Autodesk Inventor part; units mm, degrees
(part 2 of 2)
  arc A28 (126.7323, -21.9876) -> (127.2532, -22.5367) centre (141.5, -8.5) ccw projected
  spline S25 degree 3 poles (129.1537, -24.2343) (129.1768, -24.1247) (129.2231, -23.9054) (129.3093, -23.5804) (129.3922, -23.3127) (129.4667, -23.1013) (129.5266, -22.9443) (129.5917, -22.7893) (129.6822, -22.5842) (129.7847, -22.4159) (129.8454, -22.2589) (129.8618, -22.1906) (129.8689, -22.135) (129.8697, -22.0929) (129.8675, -22.0509) (129.8611, -22.0093) (129.8504, -21.9686) (129.8355, -21.9293) (129.8175, -21.8911) (129.7936, -21.8565) (129.7686, -21.8226) (129.728, -21.7839) (129.675, -21.7381) (129.6236, -21.6906) (129.5805, -21.6546) (129.544, -21.6335) (129.5069, -21.6137) (129.467, -21.6001) (129.4263, -21.5897) (129.3846, -21.5837) (129.3426, -21.5819) (129.3006, -21.5846) (129.2589, -21.5901) (129.2044, -21.6033) (129.1384, -21.6273) (128.9892, -21.7053) (128.8335, -21.826) (128.6398, -21.9391) (128.4932, -22.0211) (128.3438, -22.0983) (128.1422, -22.1961) (127.8855, -22.3086) (127.5723, -22.4308) (127.3595, -22.5014) (127.2532, -22.5367) knots 0 0 0 0 0.033613 0.067227 0.100839 0.117647 0.134454 0.151261 0.168068 0.201677 0.210077 0.218473 0.222676 0.226878 0.231076 0.235279 0.239479 0.24368 0.247882 0.252083 0.256283 0.260485 0.268889 0.277292 0.281494 0.285694 0.289895 0.294097 0.298298 0.302498 0.306701 0.310899 0.315101 0.319304 0.3277 0.3361 0.369709 0.386516 0.403323 0.420131 0.436938 0.470551 0.504164 0.537777 0.537777 0.537777 0.537777 projected
  arc A29 (129.1537, -24.2343) -> (129.7579, -24.6902) centre (141.5, -8.5) ccw projected
  spline S26 degree 3 poles (131.9119, -26.0519) (131.9167, -25.9399) (131.9262, -25.716) (131.9577, -25.3812) (131.9954, -25.1035) (132.0341, -24.8828) (132.0674, -24.718) (132.106, -24.5544) (132.1616, -24.3372) (132.235, -24.1544) (132.269, -23.9895) (132.274, -23.9194) (132.2718, -23.8634) (132.2656, -23.8218) (132.2566, -23.7807) (132.2434, -23.7408) (132.2262, -23.7023) (132.205, -23.666) (132.181, -23.6314) (132.1517, -23.6012) (132.1215, -23.5719) (132.075, -23.5403) (132.0152, -23.5039) (131.9567, -23.4655) (131.9082, -23.4371) (131.8688, -23.4223) (131.8289, -23.4088) (131.7873, -23.402) (131.7454, -23.3984) (131.7033, -23.3994) (131.6616, -23.4046) (131.6206, -23.4141) (131.5804, -23.4263) (131.5288, -23.4484) (131.4676, -23.4829) (131.3333, -23.5844) (131.1996, -23.7291) (131.0272, -23.8725) (130.8961, -23.9776) (130.7615, -24.0783) (130.5787, -24.2079) (130.344, -24.3611) (130.0551, -24.5332) (129.857, -24.6379) (129.7579, -24.6902) knots 0 0 0 0 0.033613 0.067227 0.100839 0.117647 0.134454 0.151261 0.168068 0.201677 0.210077 0.218473 0.222676 0.226878 0.231076 0.235279 0.239479 0.24368 0.247882 0.252083 0.256283 0.260485 0.268889 0.277292 0.281494 0.285694 0.289895 0.294097 0.298298 0.302498 0.306701 0.310899 0.315101 0.319304 0.3277 0.3361 0.369709 0.386516 0.403323 0.420131 0.436938 0.470551 0.504164 0.537777 0.537777 0.537777 0.537777 projected
  arc A30 (131.9119, -26.0519) -> (132.5828, -26.4021) centre (141.5, -8.5) ccw projected
  spline S27 degree 3 poles (134.9316, -27.3906) (134.9179, -27.2794) (134.8904, -27.057) (134.8664, -26.7216) (134.8579, -26.4415) (134.8597, -26.2174) (134.8654, -26.0494) (134.8766, -25.8817) (134.8957, -25.6583) (134.9379, -25.4659) (134.9444, -25.2976) (134.9378, -25.2277) (134.9264, -25.1728) (134.9134, -25.1328) (134.8978, -25.0937) (134.8782, -25.0565) (134.8549, -25.0214) (134.828, -24.9891) (134.7986, -24.9589) (134.7648, -24.9339) (134.7301, -24.91) (134.6791, -24.8865) (134.6141, -24.8604) (134.5501, -24.8322) (134.4976, -24.8121) (134.4563, -24.804) (134.4147, -24.7973) (134.3726, -24.7974) (134.3307, -24.8008) (134.2893, -24.8086) (134.249, -24.8206) (134.2101, -24.8368) (134.1725, -24.8555) (134.1252, -24.8857) (134.0706, -24.9298) (133.9548, -25.0521) (133.8467, -25.2168) (133.7003, -25.3866) (133.5882, -25.5118) (133.472, -25.6333) (133.3131, -25.7913) (133.1068, -25.981) (132.8502, -26.1983) (132.672, -26.3341) (132.5828, -26.4021) knots 0 0 0 0 0.033613 0.067227 0.100839 0.117647 0.134454 0.151261 0.168068 0.201677 0.210077 0.218473 0.222676 0.226878 0.231076 0.235279 0.239479 0.24368 0.247882 0.252083 0.256283 0.260485 0.268889 0.277292 0.281494 0.285694 0.289895 0.294097 0.298298 0.302498 0.306701 0.310899 0.315101 0.319304 0.3277 0.3361 0.369709 0.386516 0.403323 0.420131 0.436938 0.470551 0.504164 0.537777 0.537777 0.537777 0.537777 projected
  arc A31 (134.9316, -27.3906) -> (135.651, -27.6256) centre (141.5, -8.5) ccw projected
  spline S28 degree 3 poles (138.1305, -28.2141) (138.0986, -28.1067) (138.0349, -27.8918) (137.956, -27.5649) (137.9016, -27.29) (137.8665, -27.0687) (137.8445, -26.902) (137.8279, -26.7348) (137.8099, -26.5113) (137.8199, -26.3145) (137.7986, -26.1475) (137.7806, -26.0797) (137.7603, -26.0274) (137.7409, -25.99) (137.7191, -25.9541) (137.6936, -25.9206) (137.6648, -25.8898) (137.633, -25.8623) (137.5991, -25.8374) (137.5616, -25.8183) (137.5234, -25.8004) (137.4692, -25.7857) (137.4009, -25.7707) (137.333, -25.7534) (137.278, -25.7422) (137.2359, -25.741) (137.1938, -25.7412) (137.1523, -25.7482) (137.1115, -25.7585) (137.072, -25.773) (137.0342, -25.7915) (136.9985, -25.8138) (136.9644, -25.8385) (136.9228, -25.8761) (136.8762, -25.9286) (136.7821, -26.0682) (136.7026, -26.2485) (136.5861, -26.4401) (136.4962, -26.582) (136.4016, -26.721) (136.2708, -26.903) (136.0986, -27.1241) (135.8812, -27.3806) (135.7278, -27.544) (135.651, -27.6256) knots 0 0 0 0 0.033613 0.067227 0.100839 0.117647 0.134454 0.151261 0.168068 0.201677 0.210077 0.218473 0.222676 0.226878 0.231076 0.235279 0.239479 0.24368 0.247882 0.252083 0.256283 0.260485 0.268889 0.277292 0.281494 0.285694 0.289895 0.294097 0.298298 0.302498 0.306701 0.310899 0.315101 0.319304 0.3277 0.3361 0.369709 0.386516 0.403323 0.420131 0.436938 0.470551 0.504164 0.537777 0.537777 0.537777 0.537777 projected
  arc A32 (138.1305, -28.2141) -> (138.8788, -28.3275) centre (141.5, -8.5) ccw projected
  spline S29 degree 3 poles (141.4213, -28.4998) (141.3722, -28.3991) (141.274, -28.1976) (141.1424, -27.8882) (141.0434, -27.6261) (140.9724, -27.4135) (140.9232, -27.2527) (140.8793, -27.0905) (140.8248, -26.873) (140.8023, -26.6773) (140.7538, -26.5161) (140.7248, -26.4521) (140.6962, -26.4039) (140.6709, -26.3702) (140.6435, -26.3384) (140.6129, -26.3095) (140.5794, -26.2839) (140.5435, -26.262) (140.5059, -26.243) (140.4658, -26.2304) (140.4252, -26.219) (140.3693, -26.2134) (140.2994, -26.2098) (140.2297, -26.2039) (140.1735, -26.2019) (140.1318, -26.2077) (140.0904, -26.2148) (140.0505, -26.2286) (140.012, -26.2455) (139.9754, -26.2663) (139.9412, -26.2907) (139.9097, -26.3186) (139.8801, -26.3485) (139.8453, -26.3925) (139.8079, -26.452) (139.7381, -26.6052) (139.6893, -26.7961) (139.606, -27.0042) (139.5406, -27.159) (139.4702, -27.3117) (139.3711, -27.5127) (139.2377, -27.7591) (139.0655, -28.0479) (138.941, -28.2343) (138.8788, -28.3275) knots 0 0 0 0 0.033613 0.067227 0.100839 0.117647 0.134454 0.151261 0.168068 0.201677 0.210077 0.218473 0.222676 0.226878 0.231076 0.235279 0.239479 0.24368 0.247882 0.252083 0.256283 0.260485 0.268889 0.277292 0.281494 0.285694 0.289895 0.294097 0.298298 0.302498 0.306701 0.310899 0.315101 0.319304 0.3277 0.3361 0.369709 0.386516 0.403323 0.420131 0.436938 0.470551 0.504164 0.537777 0.537777 0.537777 0.537777 projected
  arc A33 (141.4213, -28.4998) -> (142.178, -28.4885) centre (141.5, -8.5) ccw projected
  spline S30 degree 3 poles (144.7142, -28.24) (144.6492, -28.1488) (144.5192, -27.9662) (144.3384, -27.6826) (144.1977, -27.4404) (144.0926, -27.2424) (144.0177, -27.0919) (143.9477, -26.9391) (143.8581, -26.7336) (143.8037, -26.5442) (143.7293, -26.3932) (143.6902, -26.3348) (143.654, -26.292) (143.6236, -26.2629) (143.5913, -26.236) (143.5563, -26.2126) (143.5191, -26.1929) (143.4801, -26.1772) (143.4399, -26.1646) (143.3982, -26.1588) (143.3563, -26.1542) (143.3003, -26.1579) (143.2307, -26.1659) (143.161, -26.1715) (143.1053, -26.1788) (143.0651, -26.1914) (143.0254, -26.2052) (142.9883, -26.2254) (142.9531, -26.2483) (142.9204, -26.2749) (142.8907, -26.3047) (142.8642, -26.3373) (142.84, -26.3717) (142.8128, -26.4208) (142.7858, -26.4856) (142.7421, -26.6482) (142.7255, -26.8446) (142.6775, -27.0636) (142.6385, -27.227) (142.5942, -27.3892) (142.5296, -27.6038) (142.4385, -27.8688) (142.3162, -28.182) (142.2241, -28.3863) (142.178, -28.4885) knots 0 0 0 0 0.033613 0.067227 0.100839 0.117647 0.134454 0.151261 0.168068 0.201677 0.210077 0.218473 0.222676 0.226878 0.231076 0.235279 0.239479 0.24368 0.247882 0.252083 0.256283 0.260485 0.268889 0.277292 0.281494 0.285694 0.289895 0.294097 0.298298 0.302498 0.306701 0.310899 0.315101 0.319304 0.3277 0.3361 0.369709 0.386516 0.403323 0.420131 0.436938 0.470551 0.504164 0.537777 0.537777 0.537777 0.537777 projected
  arc A34 (144.7142, -28.24) -> (145.4588, -28.1043) centre (141.5, -8.5) ccw projected
  spline S31 degree 3 poles (147.9195, -27.4418) (147.8403, -27.3624) (147.6821, -27.2038) (147.4571, -26.9538) (147.2784, -26.738) (147.1421, -26.56) (147.0434, -26.424) (146.9493, -26.2847) (146.8271, -26.0968) (146.7423, -25.9189) (146.644, -25.7822) (146.5958, -25.7311) (146.5531, -25.6948) (146.5183, -25.6711) (146.482, -25.6499) (146.4437, -25.6326) (146.4037, -25.6192) (146.3627, -25.6102) (146.3209, -25.6044) (146.2788, -25.6055) (146.2368, -25.6079) (146.1821, -25.6207) (146.1148, -25.6401) (146.047, -25.6571) (145.9932, -25.6735) (145.9557, -25.6925) (145.9187, -25.7127) (145.8855, -25.7387) (145.8546, -25.7671) (145.8267, -25.7987) (145.8023, -25.8329) (145.7815, -25.8695) (145.7633, -25.9074) (145.7446, -25.9603) (145.7286, -26.0287) (145.7123, -26.1963) (145.7282, -26.3927) (145.7169, -26.6166) (145.7054, -26.7842) (145.6883, -26.9515) (145.6599, -27.1738) (145.6137, -27.4501) (145.5446, -27.7792) (145.4874, -27.9959) (145.4588, -28.1043) knots 0 0 0 0 0.033613 0.067227 0.100839 0.117647 0.134454 0.151261 0.168068 0.201677 0.210077 0.218473 0.222676 0.226878 0.231076 0.235279 0.239479 0.24368 0.247882 0.252083 0.256283 0.260485 0.268889 0.277292 0.281494 0.285694 0.289895 0.294097 0.298298 0.302498 0.306701 0.310899 0.315101 0.319304 0.3277 0.3361 0.369709 0.386516 0.403323 0.420131 0.436938 0.470551 0.504164 0.537777 0.537777 0.537777 0.537777 projected
  arc A35 (147.9195, -27.4418) -> (148.6315, -27.1853) centre (141.5, -8.5) ccw projected
  spline S32 degree 3 poles (150.9496, -26.1268) (150.8585, -26.0616) (150.6763, -25.9311) (150.4132, -25.7216) (150.2014, -25.5382) (150.0378, -25.3851) (149.918, -25.2671) (149.8022, -25.1453) (149.6508, -24.98) (149.5378, -24.8185) (149.4184, -24.6998) (149.3625, -24.6574) (149.3144, -24.6286) (149.2761, -24.611) (149.2368, -24.596) (149.1962, -24.5852) (149.1546, -24.5786) (149.1126, -24.5765) (149.0705, -24.5776) (149.0291, -24.5856) (148.9881, -24.5949) (148.9362, -24.6166) (148.8731, -24.6467) (148.8089, -24.6747) (148.7586, -24.6997) (148.7247, -24.7247) (148.6916, -24.7506) (148.6631, -24.7817) (148.6372, -24.8149) (148.615, -24.8506) (148.5965, -24.8884) (148.5821, -24.9279) (148.5703, -24.9683) (148.5606, -25.0235) (148.556, -25.0936) (148.5675, -25.2616) (148.6155, -25.4527) (148.6413, -25.6754) (148.6575, -25.8427) (148.6682, -26.0104) (148.6768, -26.2344) (148.6767, -26.5146) (148.6627, -26.8506) (148.6419, -27.0737) (148.6315, -27.1853) knots 0 0 0 0 0.033613 0.067227 0.100839 0.117647 0.134454 0.151261 0.168068 0.201677 0.210077 0.218473 0.222676 0.226878 0.231076 0.235279 0.239479 0.24368 0.247882 0.252083 0.256283 0.260485 0.268889 0.277292 0.281494 0.285694 0.289895 0.294097 0.298298 0.302498 0.306701 0.310899 0.315101 0.319304 0.3277 0.3361 0.369709 0.386516 0.403323 0.420131 0.436938 0.470551 0.504164 0.537777 0.537777 0.537777 0.537777 projected
  arc A36 (150.9496, -26.1268) -> (151.6098, -25.7567) centre (141.5, -8.5) ccw projected
  spline S33 degree 3 poles (153.722, -24.331) (153.6214, -24.2817) (153.4202, -24.183) (153.1263, -24.0197) (152.8871, -23.8736) (152.7005, -23.7495) (152.563, -23.6528) (152.4287, -23.5517) (152.2521, -23.4136) (152.1141, -23.273) (151.9768, -23.1755) (151.9147, -23.1429) (151.8625, -23.1224) (151.8219, -23.1113) (151.7806, -23.103) (151.7387, -23.0991) (151.6966, -23.0994) (151.6549, -23.1042) (151.6135, -23.1123) (151.5741, -23.127) (151.5351, -23.1429) (151.4875, -23.1728) (151.4302, -23.2129) (151.3715, -23.2511) (151.326, -23.284) (151.2966, -23.3142) (151.2683, -23.3453) (151.2453, -23.3807) (151.2252, -23.4176) (151.2092, -23.4565) (151.1972, -23.4969) (151.1894, -23.5382) (151.1845, -23.58) (151.184, -23.636) (151.191, -23.7059) (151.23, -23.8697) (151.3088, -24.0503) (151.3709, -24.2657) (151.4144, -24.4281) (151.4526, -24.5918) (151.4979, -24.8113) (151.5439, -25.0877) (151.5854, -25.4214) (151.6017, -25.6449) (151.6098, -25.7567) knots 0 0 0 0 0.033613 0.067227 0.100839 0.117647 0.134454 0.151261 0.168068 0.201677 0.210077 0.218473 0.222676 0.226878 0.231076 0.235279 0.239479 0.24368 0.247882 0.252083 0.256283 0.260485 0.268889 0.277292 0.281494 0.285694 0.289895 0.294097 0.298298 0.302498 0.306701 0.310899 0.315101 0.319304 0.3277 0.3361 0.369709 0.386516 0.403323 0.420131 0.436938 0.470551 0.504164 0.537777 0.537777 0.537777 0.537777 projected
  arc A37 (153.722, -24.331) -> (154.3123, -23.8573) centre (141.5, -8.5) ccw projected
  spline S34 degree 3 poles (156.161, -22.1034) (156.0537, -22.0713) (155.839, -22.0071) (155.5221, -21.8944) (155.2622, -21.7897) (155.0578, -21.698) (154.9062, -21.6253) (154.7571, -21.5476) (154.5602, -21.4405) (154.4009, -21.3245) (154.2495, -21.251) (154.1828, -21.229) (154.1279, -21.2173) (154.086, -21.2131) (154.044, -21.2117) (154.002, -21.2147) (153.9606, -21.222) (153.9201, -21.2336) (153.8807, -21.2484) (153.8442, -21.2694) (153.8084, -21.2915) (153.7664, -21.3288) (153.7164, -21.3778) (153.6648, -21.4251) (153.6254, -21.4651) (153.6014, -21.4997) (153.5785, -21.535) (153.5617, -21.5737) (153.548, -21.6134) (153.5385, -21.6545) (153.5333, -21.6962) (153.5325, -21.7383) (153.5345, -21.7803) (153.5432, -21.8357) (153.5616, -21.9035) (153.6271, -22.0586) (153.7345, -22.2237) (153.8312, -22.426) (153.9008, -22.579) (153.9655, -22.7342) (154.0462, -22.9432) (154.1371, -23.2083) (154.233, -23.5306) (154.2858, -23.7484) (154.3123, -23.8573) knots 0 0 0 0 0.033613 0.067227 0.100839 0.117647 0.134454 0.151261 0.168068 0.201677 0.210077 0.218473 0.222676 0.226878 0.231076 0.235279 0.239479 0.24368 0.247882 0.252083 0.256283 0.260485 0.268889 0.277292 0.281494 0.285694 0.289895 0.294097 0.298298 0.302498 0.306701 0.310899 0.315101 0.319304 0.3277 0.3361 0.369709 0.386516 0.403323 0.420131 0.436938 0.470551 0.504164 0.537777 0.537777 0.537777 0.537777 projected
  arc A38 (156.161, -22.1034) -> (156.6652, -21.539) centre (141.5, -8.5) ccw projected
  spline S35 degree 3 poles (158.2001, -19.5048) (158.089, -19.4908) (157.8666, -19.4628) (157.5355, -19.4037) (157.262, -19.3432) (157.0452, -19.2864) (156.8837, -19.2397) (156.7239, -19.1876) (156.512, -19.1143) (156.3358, -19.0261) (156.1743, -18.9786) (156.1049, -18.9678) (156.0489, -18.9654) (156.0069, -18.9681) (155.9652, -18.9737) (155.9243, -18.9836) (155.8846, -18.9976) (155.8466, -19.0156) (155.8101, -19.0367) (155.7776, -19.0634) (155.7459, -19.0911) (155.7106, -19.1349) (155.6694, -19.1914) (155.6263, -19.2466) (155.594, -19.2925) (155.576, -19.3306) (155.5593, -19.3692) (155.549, -19.4101) (155.542, -19.4516) (155.5395, -19.4936) (155.5412, -19.5356) (155.5473, -19.5772) (155.5562, -19.6183) (155.5739, -19.6716) (155.6033, -19.7354) (155.6933, -19.8776) (155.8265, -20.0228) (155.9551, -20.2064) (156.049, -20.3458) (156.1383, -20.4883) (156.2524, -20.6812) (156.3857, -20.9277) (156.5333, -21.2298) (156.6213, -21.4359) (156.6652, -21.539) knots 0 0 0 0 0.033613 0.067227 0.100839 0.117647 0.134454 0.151261 0.168068 0.201677 0.210077 0.218473 0.222676 0.226878 0.231076 0.235279 0.239479 0.24368 0.247882 0.252083 0.256283 0.260485 0.268889 0.277292 0.281494 0.285694 0.289895 0.294097 0.298298 0.302498 0.306701 0.310899 0.315101 0.319304 0.3277 0.3361 0.369709 0.386516 0.403323 0.420131 0.436938 0.470551 0.504164 0.537777 0.537777 0.537777 0.537777 projected
  arc A39 (158.2001, -19.5048) -> (158.6046, -18.8651) centre (141.5, -8.5) ccw projected
  spline S36 degree 3 poles (159.7837, -16.6059) (159.6717, -16.6104) (159.4478, -16.6194) (159.1115, -16.6157) (158.8317, -16.601) (158.6085, -16.5807) (158.4416, -16.5611) (158.2754, -16.5361) (158.0543, -16.4987) (157.866, -16.4407) (157.6989, -16.4203) (157.6287, -16.4212) (157.573, -16.428) (157.532, -16.4376) (157.4918, -16.45) (157.4531, -16.4664) (157.4162, -16.4868) (157.3818, -16.5108) (157.3492, -16.5376) (157.3215, -16.5693) (157.2949, -16.6019) (157.2673, -16.6508) (157.2359, -16.7134) (157.2025, -16.7749) (157.1781, -16.8255) (157.1667, -16.866) (157.1565, -16.9069) (157.1531, -16.9489) (157.1531, -16.9909) (157.1575, -17.0328) (157.1661, -17.074) (157.179, -17.114) (157.1945, -17.1531) (157.2207, -17.2027) (157.2602, -17.2608) (157.3725, -17.3863) (157.5277, -17.5076) (157.6848, -17.6675) (157.8004, -17.7896) (157.9119, -17.9154) (158.0562, -18.0869) (158.2282, -18.3081) (158.4235, -18.5818) (158.5442, -18.7706) (158.6046, -18.8651) knots 0 0 0 0 0.033613 0.067227 0.100839 0.117647 0.134454 0.151261 0.168068 0.201677 0.210077 0.218473 0.222676 0.226878 0.231076 0.235279 0.239479 0.24368 0.247882 0.252083 0.256283 0.260485 0.268889 0.277292 0.281494 0.285694 0.289895 0.294097 0.298298 0.302498 0.306701 0.310899 0.315101 0.319304 0.3277 0.3361 0.369709 0.386516 0.403323 0.420131 0.436938 0.470551 0.504164 0.537777 0.537777 0.537777 0.537777 projected
  arc A40 (159.7837, -16.6059) -> (160.0773, -15.9084) centre (141.5, -8.5) ccw projected
  spline S37 degree 3 poles (160.8685, -13.486) (160.7588, -13.5089) (160.5394, -13.5546) (160.2071, -13.6062) (159.9287, -13.6378) (159.7052, -13.6545) (159.5373, -13.6627) (159.3693, -13.6654) (159.1451, -13.6648) (158.9498, -13.6386) (158.7816, -13.6461) (158.7125, -13.6585) (158.6587, -13.6744) (158.6199, -13.6906) (158.5822, -13.7094) (158.5467, -13.732) (158.5137, -13.7581) (158.4837, -13.7875) (158.456, -13.8193) (158.4339, -13.8551) (158.413, -13.8916) (158.3938, -13.9444) (158.3732, -14.0113) (158.3503, -14.0775) (158.3346, -14.1314) (158.33, -14.1733) (158.3267, -14.2152) (158.3303, -14.2572) (158.3372, -14.2987) (158.3484, -14.3393) (158.3637, -14.3785) (158.383, -14.4159) (158.4047, -14.4519) (158.4388, -14.4965) (158.4872, -14.5473) (158.6186, -14.6526) (158.7917, -14.7467) (158.973, -14.8786) (159.1071, -14.9799) (159.2378, -15.0857) (159.4083, -15.2311) (159.6144, -15.4209) (159.8521, -15.6587) (160.0022, -15.8252) (160.0773, -15.9084) knots 0 0 0 0 0.033613 0.067227 0.100839 0.117647 0.134454 0.151261 0.168068 0.201677 0.210077 0.218473 0.222676 0.226878 0.231076 0.235279 0.239479 0.24368 0.247882 0.252083 0.256283 0.260485 0.268889 0.277292 0.281494 0.285694 0.289895 0.294097 0.298298 0.302498 0.306701 0.310899 0.315101 0.319304 0.3277 0.3361 0.369709 0.386516 0.403323 0.420131 0.436938 0.470551 0.504164 0.537777 0.537777 0.537777 0.537777 projected
  arc A41 (160.8685, -13.486) -> (161.0433, -12.7496) centre (141.5, -8.5) ccw projected
  circle A42 centre (141.5, -8.5) radius 16 projected
  circle A43 centre (163.5, -3) radius 3
  circle A44 centre (163.5, -3) radius 1.6
  point P0 (75.5, 0)
  dimension "d56" = 6
  dimension "d57" = 3.2
  dimension "d58" = 3
  dimension "d59" = 3
  constraints: 2 centre point, 1 coincident
  measures "d56" diameter of A43
  measures "d57" diameter of A44
  measures "d58" distance from line of L2 A44.centre
  measures "d59" distance from line of L1 A43.centre
hole "Hole3" at (88, 34, 3) direction (0, -1, 0) diameter 3.6 end through all countersink diameter 6 countersink angle 90
mirror "Mirror1" about plane through (0, 0, 0) normal (0, 1, 0) remove original yes
ref_plane "Work Plane2" through (-36.05, -52.6, 20.5) normal (-1, 0, 0) x (0, -1, 0)
sketch "Sketch15" plane through (-36.05, -52.6, 20.5) normal (-1, 0, 0) x (0, -1, 0)
  line L0 (0, -0.8) -> (-18.6, -0.8)
  line L1 (-18.6, -9.3605) -> (-18.6, 9.5) projected
  line L2 (-18.6, -13.1659) -> (-18.6, -9.3605)
  line L3 (-18.6, -13.1659) -> (-6.2341, -0.8)
  point P0 (-52.6, -20.5)
  dimension "d75" = 45
  constraints: 6 end point, 2 point on line, 1 collinear, 1 horizontal, 2 other
  measures "d75" angle of L0 L3
extrude "Extrusion13" add sketch "Sketch15" against normal blind 8
ref_plane "Work Plane3" through (5.25, -34, 20.5) normal (1, 0, 0) x (0, 1, 0)
sketch "Sketch16" plane through (5.25, -34, 20.5) normal (1, 0, 0) x (0, 1, 0)
  line L0 (0, -17.5) -> (0, 9.5) projected
  line L1 (0, -0.8) -> (-18.6, -0.8)
  line L2 (-18.6, -0.8) -> (0, -19.4)
  line L3 (0, -19.4) -> (0, -17.5)
  point P0 (34, -20.5)
  dimension "d78" = 45
  constraints: 6 end point, 1 horizontal, 1 point on line, 1 vertical, 2 other
  measures "d78" angle of L1 L2
extrude "Extrusion14" add sketch "Sketch16" against normal blind 8
sketch "Sketch17" plane through (-36.05, -46.3659, 19.7) normal (0, 0, 1) x (1, 0, 0)
  circle A0 centre (3.45, 9.0659) radius 1.5
  circle A1 centre (37.85, 9.0659) radius 1.5
  point P0 (36.05, 46.3659)
  constraints: 2 centre point, 2 coincident, 4 other
hole "Hole4" at (-32.6, -37.3, 19.7) at (1.8, -37.3, 19.7) direction (0, 0, -1) diameter 4 depth 5.8 counterbore diameter 4.6 counterbore depth 1.3
sketch "Sketch18" plane through (10.65, -32, 30) normal (-1, 0, 0) x (0, 0, 1)
  line L0 (-15.5, 0) -> (-15.5, 5) projected
  line L1 (-15.5, 5) -> (-15.5, 12)
  line L2 (-15.5, 12) -> (-23.7583, 3.7417)
  line L3 (-15.5, 5) -> (-30, 5)
  point P0 (-30, 32)
  point P1 (-22.5, 5)
  dimension "d88" = 45
  dimension "d92" = 12
  constraints: 6 end point, 1 vertical
  measures "d88" angle of L1 L2
  measures "d92" distance of L1.end L0.start
extrude "Extrusion15" add sketch "Sketch18" along normal up to surface (16.8 mm away)
equation "\"d58\" = 0.5 * d56"
equation "\"d59\" = 0.5 * d56"
body "Solid1"
